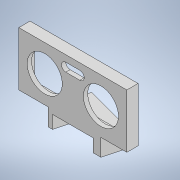
# Autodesk Inventor part: Крепление ультрасоника вертикальная
Saved by Autodesk Inventor 2020 (Build 240168000, 168)
## iProperties
Created: 2021-05-10
Part Number: Крепление ультрасоника вертикальная
Material: Типовые
Document SubType Name: Modeling
Designer: Антон
Density: 1 g/cm^3
Appearance: По умолчанию
Author: Антон
Autodesk Inventor part; units mm, degrees
note: some values were not read from the file. Chosen so that the rebuilt part matches the saved one: direction of "Отверстие4".
ref_plane "YZ Plane" through (0, 0, 0) normal (1, 0, 0) x (0, 1, 0)
sketch "Эскиз1" plane through (0, 0, 0) normal (0, 0, 1) x (1, 0, 0)
  line L0 (0, 0) -> (50, 0)
  line L1 (50, 0) -> (50, 25)
  line L2 (50, 25) -> (0, 25)
  line L3 (0, 25) -> (0, 0)
  dimension "d0" = 50
  dimension "d1" = 25
  constraints: 8 end point, 2 parallel, 1 horizontal, 1 perpendicular
  measures "d0" distance of L2.end L1.end
  measures "d1" distance of L1.end L0.end
extrude "Выдавливание1" add sketch "Эскиз1" along normal blind 5.2
shell "Оболочка1" thickness 2 removed faces 1 at (16.6667, 16.6667, 0)
sketch "Эскиз2" plane through (0, 0, 5.2) normal (0, 0, 1) x (1, 0, 0)
  line L0 (50, 25) -> (0, 25) projected
  line L1 (25, 25) -> (25, 0)
  line L2 (0, 0) -> (50, 0) projected
  line L3 (25, 12.5) -> (12, 12.5)
  line L4 (0, 25) -> (0, 0) projected
  circle A0 centre (12, 12.5) radius 8.1
  circle A1 centre (38, 12.5) radius 8.1
  line L5 (25, 25) -> (25, 20)
  line L6 (21.75, 20) -> (28.25, 20) construction
  line L7 (21.75, 18) -> (28.25, 18)
  line L8 (28.25, 22) -> (21.75, 22)
  arc A2 (21.75, 22) -> (21.75, 18) centre (21.75, 20) ccw
  arc A3 (28.25, 18) -> (28.25, 22) centre (28.25, 20) ccw
  point P0 (25, 18)
  point P1 (25, 22)
  dimension "d5" = 13
  dimension "d6" = 16.2
  dimension "d9" = 5
  dimension "d10" = 3.25
  dimension "d11" = 4
  constraints: 14 end point, 4 centre point, 4 midpoint, 4 point on circle, 4 tangent, 1 coincident, 1 horizontal, 1 parallel, 1 perpendicular, 1 point on line, 1 symmetric about line, 1 other
  measures "d5" distance of L3.start L3.end
  measures "d6" diameter of A0
  measures "d9" distance of L1.start L5.end
  measures "d10" distance of L5.end L6.end
  measures "d11" diameter of A3
extrude "Выдавливание2" cut sketch "Эскиз2" against normal through all contours L8 A3 L7 L1 | L1 L7 A2 L8 | A0 | A1
sketch "Эскиз5" plane through (48, 23, 3.2) normal (0, 0, -1) x (-1, 0, 0)
  line L0 (0, 0) -> (1.05, 0)
  line L1 (0, 0) -> (46, 0) projected
  line L2 (1.05, 0) -> (1.05, -1.05)
  circle A0 centre (1.05, -1.05) radius 1.05
  line L3 (2.1, -2.1) -> (0, -2.1)
  line L4 (0, -2.1) -> (0, 0)
  line L5 (0, 0) -> (2.1, 0)
  line L6 (2.1, 0) -> (2.1, -2.1)
  line L7 (2.1, -2.1) -> (0, 0) construction
  line L8 (0, -2.1) -> (2.1, 0) construction
  point P0 (48, -23)
  point P1 (1.05, -2.1)
  point P2 (2.1, -1.05)
  dimension "d17" = 1.05
  dimension "d18" = 1.05
  constraints: 16 end point, 2 midpoint, 2 parallel, 1 coincident, 1 horizontal, 1 perpendicular, 1 point on line, 1 vertical, 3 other
  measures "d17" distance of L0.start L0.end
  measures "d18" distance of L0.end L2.end
extrude "Выдавливание4" add sketch "Эскиз5" along normal blind 1 contours L0 A0 L4 | L1 L6 A0 | A0 | A0 L3 L4
ref_plane "РабПлоскость1" through (25, 2, 0) normal (1, 0, 0) x (0, 0, -1)
ref_plane "РабПлоскость2" through (2, 12.5, 0) normal (0, -1, 0) x (1, 0, 0)
mirror "Зеркальное отражение1" about plane through (2, 12.5, 0) normal (0, -1, 0) of "Выдавливание4"
mirror "Зеркальное отражение2" about plane through (25, 2, 0) normal (1, 0, 0) of "Выдавливание4", "Зеркальное отражение1"
sketch "Эскиз14" plane through (0, 0, 0) normal (0, -1, 0) x (1, 0, 0)
  line L0 (35.6735, 8.06) -> (14.3265, 2.34)
  line L1 (14.3265, 2.34) -> (17.8206, -10.6999)
  line L2 (17.8206, -10.6999) -> (39.1675, -4.98)
  line L3 (39.1675, -4.98) -> (35.6735, 8.06)
  line L4 (35.6735, 8.06) -> (17.8206, -10.6999) construction
  line L5 (14.3265, 2.34) -> (39.1675, -4.98) construction
  line L6 (0, 5.2) -> (50, 5.2) projected
  point P0 (0, 0)
  point P1 (26.747, -1.32)
  point P2 (25, 5.2)
  dimension "d67" = 13.5
  dimension "d68" = 22.1
  dimension "d77" = 15
  constraints: 12 end point, 4 midpoint, 2 parallel, 1 perpendicular
  measures "d67" distance of L2.end L0.start
  measures "d68" distance of L1.end L2.end
  measures "d77" angle of L6 L0
extrude "Выдавливание10" add sketch "Эскиз14" along normal blind 8
sketch "Эскиз15" plane through (0, -8, 0) normal (0, -1, 0) x (1, 0, 0)
  line L0 (17.8206, -10.6999) -> (39.1675, -4.98) projected
  line L1 (19.2348, -8.2505) -> (36.718, -3.5658)
  line L2 (36.718, -3.5658) -> (34.2593, 5.6105)
  line L3 (34.2593, 5.6105) -> (16.776, 0.9258)
  line L4 (16.776, 0.9258) -> (19.2348, -8.2505)
  line L5 (39.1675, -4.98) -> (35.6735, 8.06) projected
  line L6 (17.8206, -10.6999) -> (39.1675, -4.98) projected
  line L7 (35.6735, 8.06) -> (14.3265, 2.34) projected
  line L8 (39.1675, -4.98) -> (14.3265, 2.34) construction
  line L9 (17.8206, -10.6999) -> (35.6735, 8.06) construction
  line L10 (19.2348, -8.2505) -> (34.2593, 5.6105) construction
  line L11 (16.776, 0.9258) -> (36.718, -3.5658) construction
  line L12 (34.2593, 5.6105) -> (33.7416, 7.5423)
  line L13 (16.776, 0.9258) -> (16.2584, 2.8577)
  point P0 (0, 0)
  point P1 (26.747, -1.32)
  dimension "d78" = 2
  dimension "d79" = 2
  constraints: 20 end point, 3 parallel, 2 collinear, 2 midpoint, 2 point on line, 1 perpendicular
  measures "d78" distance between parallel lines of L0 L1
  measures "d79" distance between parallel lines of L5 L2
extrude "Выдавливание11" cut sketch "Эскиз15" against normal blind 6
sketch "Эскиз16" plane through (37.8331, 0, 0) normal (0.9659258, 0, 0.258819) x (0.258819, 0, -0.9659258)
  line L0 (5.1557, 0) -> (0, 0) projected
  line L1 (-5.3834, 0) -> (0, 0) projected
  line L2 (-8.3443, 0) -> (-8.3443, -8) projected
  line L3 (5.1557, -8) -> (-8.3443, -8) projected
  line L4 (5.1557, 0) -> (5.1557, -8) projected
  line L5 (-5.3834, 0) -> (-8.3443, 0) projected
  point P0 (-9.7919, 0)
extrude "Выдавливание12" add sketch "Эскиз16" along normal blind 1.5
sketch "Эскиз17" plane through (17.8206, -8, -10.6999) normal (-0.9659258, 0, -0.258819) x (-0.258819, 0, 0.9659258)
  line L0 (2, 0) -> (13.5, 0) projected
  line L1 (2, 0) -> (2, 6) projected
  line L2 (2, 6) -> (13.5, 6) projected
  line L3 (13.5, 0) -> (13.5, 6) projected
  line L4 (7.75, 6) -> (7.75, 0)
  line L5 (13.5, 0) -> (0, 0) projected
  point P0 (14.9477, 8)
  point P1 (7.75, 3)
  constraints: 2 end point, 2 midpoint, 1 perpendicular, 1 point on line
hole "Отверстие4" at (15.8147, -5, -3.214) direction (0.9659258, 0, 0.258819) diameter 2 depth 2
sketch "Эскиз18" plane through (0, 0, 0) normal (0, 1, 0) x (1, 0, 0)
  line L0 (25, -5.2) -> (37.9927, -5.2) projected
  line L1 (25, -5.2) -> (37.1224, -8.4482) projected
  line L2 (37.9927, -5.2) -> (37.1224, -8.4482) projected
  point P0 (0, 0)
extrude "Выдавливание13" cut sketch "Эскиз18" against normal through all
sketch "Эскиз19" plane through (0, 0, 0) normal (0, -1, 0) x (1, 0, 0)
  line L0 (14.3265, 2.34) -> (25, 5.2) projected
  line L1 (14.3265, 2.34) -> (13.5602, 5.2)
  line L2 (0, 5.2) -> (25, 5.2) projected
  line L3 (14.3265, 2.34) -> (17.8206, -10.6999) projected
  line L4 (16.2584, 2.8577) -> (14.3265, 2.34) projected
  line L5 (16.2584, 2.8577) -> (15.6308, 5.2)
  line L6 (50, 5.2) -> (0, 5.2) projected
  line L7 (19.2348, -8.2505) -> (16.2584, 2.8577) projected
  point P0 (0, 0)
  constraints: 4 end point, 2 collinear, 2 point on line
extrude "Выдавливание14" add sketch "Эскиз19" along normal up to surface (8 mm away) contours L1 L2 L5 L0
sketch "Эскиз21" plane through (15.6308, 0, 5.2) normal (0, -1, 0) x (1, 0, 0)
  line L0 (0, 0) -> (0.6276, -2.3423) projected
  line L1 (0.6276, -2.3423) -> (9.3692, 0) projected
  line L2 (0, 0) -> (9.3692, 0) projected
  point P0 (-15.6308, -5.2)
extrude "Выдавливание15" add sketch "Эскиз21" along normal up to surface (2 mm away)
